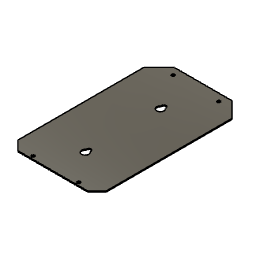
Full Cover v11 (Autodesk Fusion 360 design; units mm, degrees)
Autodesk Fusion 360 part; units mm, degrees
note: some values were not read from the file. Set by a fixed rule: which sketch regions a step uses.
sketch "Sketch1" plane through (0, 0, 0) normal (0, 0, 1) x (1, 0, 0)
  line L0 (0, 0) -> (145, 0)
  line L1 (145, 0) -> (145, 247.018)
  line L2 (145, 247.018) -> (0, 247.018)
  line L3 (0, 247.018) -> (0, 0)
  dimension "d1" = 247.018
  dimension "d2" = 145
  constraint horizontal L0
  constraint vertical L1
  constraint horizontal L2
  constraint vertical L3
  constraint coincident L0.start L3.end
  measures "d1" distance of L0.end L1.end
  measures "d2" distance of L0.start L0.end
extrude "Extrude1" add sketch "Sketch1" along normal blind 3
chamfer "Chamfer1" distance 15 angle 45 2 edges at (0, 0, 1.5) (145, 0, 1.5)
chamfer "Chamfer2" distance 25 angle 45 2 edges at (0, 247.018, 1.5) (145, 247.018, 1.5)
sketch "Sketch3" plane through (0, 0, 3) normal (0, 0, 1) x (-1, 0, 0)
  line L0 (-145, -222.018) -> (-120, -247.018)
  line L1 (-120, -247.018) -> (-25, -247.018)
  line L2 (-25, -247.018) -> (0, -222.018)
  line L3 (0, -222.018) -> (0, -15)
  line L4 (0, -15) -> (-15, 0)
  line L5 (-15, 0) -> (-130, 0)
  line L6 (-130, 0) -> (-145, -15)
  line L7 (-145, -15) -> (-145, -222.018)
  circle A0 centre (-35, -235.018) radius 2.5
  circle A1 centre (-110, -235.018) radius 2.5
  circle A2 centre (-110, -5) radius 2.5
  circle A3 centre (-35, -5) radius 2.5
  circle A4 centre (-35, -5) radius 1.65
  circle A5 centre (-110, -5) radius 1.65
  circle A6 centre (-110, -235.018) radius 1.65
  circle A7 centre (-35, -235.018) radius 1.65
  dimension "d27" = 35
  dimension "d28" = 35
  dimension "d29" = 12
  dimension "d30" = 5
  dimension "d31" = 5
  dimension "d32" = 5
  dimension "d33" = 5
  dimension "d34" = 5
  dimension "d35" = 3.3
  dimension "d36" = 3.3
  dimension "d37" = 3.3
  dimension "d38" = 3.3
  constraint horizontal A0.centre A1.centre
  constraint horizontal A2.centre A3.centre
  constraint vertical A1.centre A2.centre
  constraint vertical A0.centre A3.centre
  constraint concentric A3 A4
  constraint concentric A2 A5
  constraint concentric A1 A6
  constraint concentric A0 A7
  measures "d27" distance of L3 A0.centre
  measures "d28" distance of L7 A1.centre
  measures "d29" distance of L1 A1.centre
  measures "d30" diameter of A0
  measures "d31" diameter of A1
  measures "d32" diameter of A3
  measures "d33" diameter of A2
  measures "d34" distance of L5 A3.centre
  measures "d35" diameter of A4
  measures "d36" diameter of A5
  measures "d37" diameter of A6
  measures "d38" diameter of A7
extrude "Extrude5" cut sketch "Sketch3" against normal blind 2 contours A0 | A1 | A2 | A3
extrude "Extrude4" cut sketch "Sketch3" against normal blind 3 contours A4 | A5 | A6 | A7
sketch "Sketch4" plane through (0, 0, 3) normal (0, 0, 1) x (-1, 0, 0)
  circle A0 centre (-110, -5) radius 2.5
  circle A1 centre (-110, -235.018) radius 2.5
  circle A2 centre (-35, -5) radius 2.5
  circle A3 centre (-35, -235.018) radius 2.5
  line L0 (-145, -222.018) -> (-120, -247.018)
  line L1 (-120, -247.018) -> (-25, -247.018)
  line L2 (-25, -247.018) -> (0, -222.018)
  line L3 (0, -222.018) -> (0, -15)
  line L4 (0, -15) -> (-15, 0)
  line L5 (-15, 0) -> (-130, 0)
  line L6 (-130, 0) -> (-145, -15)
  line L7 (-145, -15) -> (-145, -222.018)
  line L8 (-72.5, -247.018) -> (-72.5, 0)
  line L9 (0, -118.509) -> (-145, -118.509)
  line L10 (-72.5, -118.509) -> (-72.5, -247.018)
  line L11 (-72.5, -182.7635) -> (0, -182.7635)
  line L12 (-72.5, -118.509) -> (-72.5, 0)
  line L13 (-72.5, -59.2545) -> (0, -59.2545)
  circle A4 centre (-72.5, -182.7635) radius 3.5
  circle A5 centre (-72.5, -59.2545) radius 3.5
  circle A6 centre (-72.5, -53.2545) radius 6
  circle A7 centre (-72.5, -176.7635) radius 6
  dimension "d43" = 7
  dimension "d44" = 7
  dimension "d45" = 12
  dimension "d46" = 12
  constraint midpoint L1 L8.start
  constraint midpoint L5 L8.end
  constraint midpoint L3 L9.start
  constraint midpoint L7 L9.end
  constraint midpoint L9 L10.start
  constraint midpoint L10 L11.start
  constraint coincident L3 L11.end
  constraint perpendicular L8 L11
  constraint midpoint L12 L13.start
  constraint coincident L3 L13.end
  constraint perpendicular L3 L13
  constraint coincident L11.start A4.centre
  constraint coincident L13.start A5.centre
  constraint coincident L12 A6.centre
  constraint coincident L13.start A6
  constraint coincident L10 A7.centre
  constraint coincident L11.start A7
  measures "d43" diameter of A4
  measures "d44" diameter of A5
  measures "d45" diameter of A6
  measures "d46" diameter of A7
extrude "Extrude6" cut sketch "Sketch4" against normal blind 3 contours L8 L12 A5 A6 | L8 L12 L13 A5 | L8 L12 A5 A6 | L13 A5 A6 | L8 L12 A5 A6 | L8 L12 A5 A6 | L8 L12 A5 A6
extrude "Extrude7" cut sketch "Sketch4" against normal blind 3 contours L8 L10 A4 A7 | L8 L10 L11 A4 | L8 L10 A4 A7 | L8 L10 A4 A7 | L8 L10 A4 A7 | L11 A4 A7 | L8 L10 A4 A7
extrude "Extrude10" cut sketch "Sketch3" against normal blind 1 contours L0 L1 L2 L3 L4 L5 L6 L7
extrude "Extrude11" cut 1 faces at (122.568, 136.9318, 0) along direction (0, 0, 1) blind 0.5
